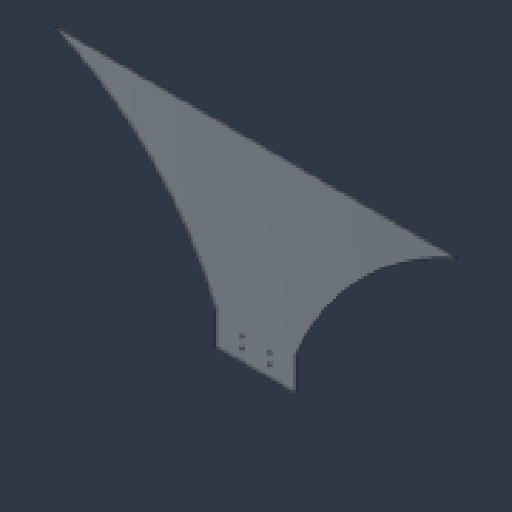
# Autodesk Inventor part: curved_hopper_back
Saved by Autodesk Inventor 2024.3 (Build 283343000, 343)
## iProperties
Created: 2025-03-30
Part Number: curved_hopper_back
Material: Polycarbonate, Clear
Document SubType Name: Sheet Metal
Designer: marcu
Density: 1.2 g/cm^3
Sheet Metal Rule: Default
Appearance: Polycarbonate - Clear
Author: marcu
Autodesk Inventor part; units mm, degrees
ref_plane "YZ Plane" through (0, 0, 0) normal (1, 0, 0) x (0, 1, 0)
ref_plane "XZ Plane" through (0, 0, 0) normal (0, 1, 0) x (-1, 0, 0)
ref_plane "XY Plane" through (0, 0, 0) normal (0, 0, 1) x (1, 0, 0)
sketch "Sketch1" plane through (0, 0, 0) normal (0, 0, 1) x (1, 0, 0)
  line L0 (70.485, -28.575) -> (-70.485, -28.575)
  line L1 (-70.485, -28.575) -> (-70.485, 28.575)
  line L2 (-70.485, 28.575) -> (70.485, 28.575)
  line L3 (70.485, 28.575) -> (70.485, -28.575)
  line L4 (70.485, -28.575) -> (-70.485, 28.575) construction
  line L5 (-70.485, -28.575) -> (70.485, 28.575) construction
  line L6 (-361.95, 327.025) -> (361.95, 327.025)
  line L7 (-361.95, 327.025) -> (-361.95, 352.425) construction
  line L8 (-70.485, 28.575) -> (-45.085, 28.575) construction
  line L9 (0, 0) -> (0, 28.575) construction
  arc A0 (-70.485, 28.575) -> (-361.95, 327.025) centre (-587.1049, -184.407) ccw
  arc A1 (361.95, 327.025) -> (70.485, 28.575) centre (587.1049, -184.407) ccw
  point P0 (0, 327.025)
  dimension "d0" = 140.97
  dimension "d1" = 57.15
  dimension "d2" = 723.9
  dimension "d3" = 355.6
  dimension "d4" = 25.4
  dimension "d7" = 558.8
  measures "d0" distance of L1.end L2.end
  measures "d1" distance of L0.end L1.end
  measures "d2" distance of L6.start L6.end
  measures "d3" distance between parallel lines of L0 L6
  measures "d4" distance of L6.start L7.end
  measures "d7" radius of A0
extrude "Plate1" add sketch "Sketch1" along normal blind 3.048
sketch "Sketch2" plane through (0, 0, 3.048) normal (0, 0, 1) x (1, 0, 0)
  line L0 (70.485, -28.575) -> (-70.485, -28.575) construction
  line L1 (-25.4, -28.575) -> (-25.4, -7.9375) construction
  point P0 (0, 0)
  point P1 (25.4, -7.9375)
  point P2 (-25.4, 11.1125)
  point P3 (25.4, 11.1125)
  dimension "d9" = 20.6375
  dimension "d11" = 25.4
  dimension "d15" = 50.8
  dimension "d18" = 19.05
  constraints: 2 end point, 1 coincident, 1 horizontal, 1 perpendicular, 1 point on line, 1 vertical, 3 other
  measures "d9" distance of L1.start L1.end
  measures "d11" distance from line of L1 point (0, 0)
  measures "d15" distance of point (-25.4, -7.937) point (25.4, -7.937)
  measures "d18" distance of point (-25.4, -7.937) point (-25.4, 11.113)
hole "Hole1" at (-25.4, -7.9375, 3.048) at (25.4, -7.9375, 3.048) at (-25.4, 11.1125, 3.048) at (25.4, 11.1125, 3.048) direction (0, 0, -1) diameter 5.1054 depth 3.048 tip angle 118 clearance for "Flat Head Machine Screw (82)" size "#10" standard "Ansi Unified Screw Threads"
sketch "Sketch3" plane through (0, 0, 0) normal (0, 0, -1) x (-1, 0, 0)
  arc A0 (361.95, 327.025) -> (70.485, 28.575) centre (587.1049, -184.407) ccw construction
  line L0 (187.323, 206.0182) -> (178.2371, 214.8915) construction
  line L1 (169.3637, 205.8056) -> (187.1104, 223.9775) construction
  line L2 (169.3637, 205.8056) -> (151.1918, 223.5522) construction
  line L3 (187.1104, 223.9775) -> (168.9384, 241.7241) construction
  line L4 (0, 0) -> (0, 25.4) construction
  point P0 (-169.3637, 205.8056)
  point P1 (-187.1104, 223.9775)
  point P2 (-151.1918, 223.5522)
  point P3 (-168.9384, 241.7241)
  dimension "d28" = 12.7
  dimension "d29" = 25.4
  dimension "d30" = 25.4
  dimension "d31" = 25.4
  dimension "d32" = 25.4
  constraints: 10 end point, 4 coincident, 4 symmetric about line, 3 perpendicular, 1 line through centre, 1 midpoint, 1 point on circle, 1 vertical
  measures "d28" distance of L0.end L0.start
  measures "d29" distance of L1.start L1.end
  measures "d30" distance of L2.start L2.end
  measures "d31" distance of L3.start L3.end
  measures "d32" distance of L4.start L4.end
hole "Hole2" at (-169.3637, 205.8056, 0) at (-187.1104, 223.9775, 0) at (-151.1918, 223.5522, 0) at (-168.9384, 241.7241, 0) at (151.1918, 223.5522, 0) at (169.3637, 205.8056, 0) at (187.1104, 223.9775, 0) at (168.9384, 241.7241, 0) direction (0, 0, 1) diameter 5.1054 depth 3.048 tip angle 118 clearance for "Flat Head Machine Screw (82)" size "#10" standard "Ansi Unified Screw Threads"
sketch "Sketch4" plane through (0, 0, 0) normal (0, 0, -1) x (-1, 0, 0)
  point P0 (0, 0)
equation "\"d26\" = Thickness"
equation "\"d38\" = Thickness"
equation "\"d8\" = Thickness"
equation "\"BendRadius\" = Thickness"
equation "\"BendReliefWidth\" = Thickness"
equation "\"BendReliefDepth\" = 0.5 * Thickness"
equation "\"CornerReliefSize\" = 4 * Thickness"
equation "\"MinimumRemnant\" = 2 * Thickness"
equation "\"TransitionRadius\" = BendRadius"
equation "\"JacobiRadiusSize\" = BendRadius"
equation "\"GapSize\" = Thickness"
equation "\"Thickness\" = 3.048"
body "Solid1"
